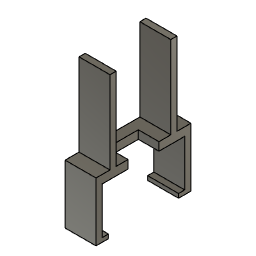
assembly v45 (Autodesk Fusion 360 archive; units mm, degrees)
design "bottom clip"
Autodesk Fusion 360 part; units mm, degrees
sketch "Sketch1" plane through (0, 0, 0) normal (1, 0, 0) x (0, 1, 0)
  line L0 (0, 0) -> (8, 0)
  line L1 (8, 0) -> (8, -9)
  line L2 (8, -9) -> (6.8, -9)
  line L3 (6.8, -9) -> (6.8, -9.8)
  line L4 (6.8, -9.8) -> (9.2, -9.8)
  line L5 (9.2, -9.8) -> (9.2, 1.6)
  line L6 (9.2, 1.6) -> (6.5, 1.6)
  line L7 (6.5, 1.6) -> (6.5, 17.6)
  line L8 (6.5, 17.6) -> (5.3, 17.6)
  line L9 (5.3, 17.6) -> (5.3, 1.6)
  line L10 (5.3, 1.6) -> (0, 1.6)
  line L11 (0, 1.6) -> (0, 0)
  dimension "d1" = 1.2
  dimension "d2" = 1.2
  dimension "d3" = 1.6
  dimension "d4" = 8
  dimension "d6" = 0.8
  dimension "d7" = 1.2
  dimension "d8" = 16
  dimension "d9" = 5.3
  dimension "d17" = 9
  constraint coincident L0.start L11.end
  constraint horizontal L0
  constraint perpendicular L0 L1
  constraint perpendicular L1 L2
  constraint perpendicular L2 L3
  constraint perpendicular L1 L4
  constraint perpendicular L4 L5
  constraint perpendicular L5 L6
  constraint perpendicular L6 L7
  constraint perpendicular L7 L8
  constraint perpendicular L6 L9
  constraint perpendicular L9 L10
  constraint perpendicular L0 L11
  constraint collinear L6 L10
  measures "d1" distance of L1 L5
  measures "d2" distance of L7 L9
  measures "d3" distance of L0 L10
  measures "d4" distance of L0.start L0.end
  measures "d6" distance of L2.end L3.end
  measures "d7" distance of L1.end L2.end
  measures "d8" distance of L6.end L7.end
  measures "d9" distance of L9.end L10.end
  measures "d17" distance of L0.end L1.end
extrude "Extrude1" add sketch "Sketch1" along normal blind 6
sketch "Sketch2" plane through (0, 0, 1.6) normal (0, 0, 1) x (-1, 0, 0)
  line L0 (0, -5.3) -> (0, 0)
  line L1 (0, 0) -> (-6, 0)
  line L2 (-6, 0) -> (-6, -5.3)
  line L3 (-6, -5.3) -> (0, -5.3)
  line L4 (-6, 0) -> (-2, 0)
  line L5 (-2, 0) -> (-2, -3)
  line L6 (-2, -3) -> (-6, -3)
  line L7 (-6, -3) -> (-6, 0)
  dimension "d12" = 4
  dimension "d13" = 3
  constraint horizontal L4
  constraint vertical L5
  constraint horizontal L6
  constraint vertical L7
  constraint coincident L1.end L2.start
  measures "d12" distance of L5.end L6.end
  measures "d13" distance of L1.end L6.end
extrude "Extrude2" cut sketch "Sketch2" against normal through all contours L1 L2 L4 L5 L6 L7
mirror "Mirror1" about plane through (0, 0, 0) normal (0, 1, 0) of bodies 1 merged

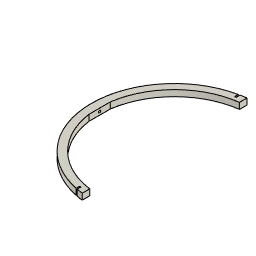
design "midRing"
Autodesk Fusion 360 part; units mm, degrees
sketch "Sketch1" plane through (0, 0, 0) normal (0, 0, 1) x (1, 0, 0)
  circle A0 centre (0, 0) radius 100
  circle A1 centre (0, 0) radius 105
  circle A2 centre (0, 0) radius 109.9
  line L0 (0, 0) -> (0, -109.9) construction
  line L1 (0, 0) -> (109.9, 0) construction
  line L2 (13, -99.1514) -> (13, -109.1284)
  line L3 (-13, -99.1514) -> (-13, -109.1284)
  circle A3 centre (-18, -103.4456) radius 1.5
  circle A4 centre (-28, -101.1978) radius 1.5
  line L4 (-13, 99.1514) -> (-13, 109.1284)
  line L5 (13, 99.1514) -> (13, 109.1284)
  circle A5 centre (-18, 103.4456) radius 1.5
  circle A6 centre (-28, 101.1978) radius 1.5
  line L6 (-22.7, -107.5301) -> (-22.7, -102.875)
  line L7 (-22.7, -102.875) -> (-21, -102.875)
  line L8 (-21, -102.875) -> (-21, -107.875)
  line L9 (-22.7, 107.5301) -> (-22.7, 102.875)
  line L10 (-21, 102.875) -> (-21, 107.875)
  line L11 (-22.7, 102.875) -> (-21, 102.875)
  line L12 (-99, 14.1067) -> (-99, -14.1067)
  line L13 (-100, 0) -> (0, 0) construction
  dimension "d1" = 200
  dimension "d2" = 5
  dimension "d3" = 9.9
  dimension "d4" = 26
  dimension "d5" = 5
  dimension "d7" = 3
  dimension "d8" = 3
  dimension "d9" = 10
  dimension "d21" = 8
  dimension "d22" = 1.7
  dimension "d23" = 5
  dimension "d24" = 1
  constraint coincident A0.centre A1.centre
  constraint concentric A0 A1
  constraint coincident A2 L0.end
  constraint vertical L0
  constraint coincident A2 L1.end
  constraint perpendicular L0 L1
  constraint coincident A0 L2.start
  constraint coincident A2 L2.end
  constraint perpendicular L1 L2
  constraint coincident A0 L3.start
  constraint coincident A2 L3.end
  constraint parallel L2 L3
  constraint equal L2 L3
  constraint coincident A1 A3.centre
  constraint coincident A1 A4.centre
  constraint symmetric L1 L2.start L5.start
  constraint symmetric L1 L2.end L5.end
  constraint symmetric L1 L3.start L4.start
  constraint symmetric L1 L3.end L4.end
  constraint symmetric L1 A3 A5
  constraint symmetric L1 A4 A6
  constraint coincident A2 L6.start
  constraint vertical L6
  constraint perpendicular L6 L7
  constraint coincident A2 L8.end
  constraint perpendicular L7 L8
  constraint symmetric L1 L6.start L9.start
  constraint symmetric L1 L6.end L9.end
  constraint symmetric L1 L7.end L10.start
  constraint symmetric L1 L8.end L10.end
  constraint coincident A0 L12.start
  constraint coincident A0 L12.end
  constraint vertical L12
  constraint coincident A0 L13.start
  constraint perpendicular L0 L13
  measures "d1" diameter of A0
  measures "d2" distance of A0 A1
  measures "d3" distance of A0 A2
  measures "d4" distance of L2 L3
  measures "d5" distance of L3 A3.centre
  measures "d7" diameter of A4
  measures "d8" diameter of A3
  measures "d9" horizontal distance of A3.centre A4.centre
  measures "d21" distance of L3 L8
  measures "d22" distance of L6.end L7.end
  measures "d23" distance of L7.end L8.end
  measures "d24" distance of L12 L13.start
extrude "Extrude1" add sketch "Sketch1" along normal mid plane 8.1 contours A0 A1 L3 A3 A4 L4 A5 A6 L7 L8 L10 L11 | A0 L12 | A1 A2 L4 A5 L10 | A1 A2 L3 A3 L8 | A1 A5 | A1 A5 | A1 A3 | A1 A3 | A1 A2 A4 A6 L6 L7 L9 L11 | A1 A6 | A1 A6 | A1 A4 | A1 A4 picked at (-99.2962, 1.5721)
ref_plane "WorkPlane1" through (-110, 0, 0) normal (1, 0, 0) x (0, 1, 0)
sketch "Sketch3" plane through (-110, 0, 0) normal (1, 0, 0) x (0, 1, 0)
  circle A0 centre (0, 0) radius 1.55
  dimension "d16" = 3.1
  constraint coincident A0.centre origin
  measures "d16" diameter of A0
extrude "Extrude4" cut sketch "Sketch3" along normal through all

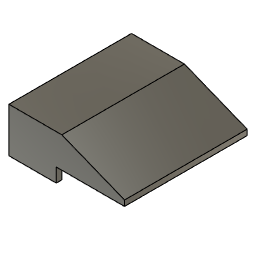
design "top clip"
Autodesk Fusion 360 part; units mm, degrees
sketch "Sketch1" plane through (0, 0, 0) normal (0, 0, 1) x (1, 0, 0)
  line L0 (3, 8) -> (-3, 8)
  line L1 (-3, 8) -> (-3, -8)
  line L2 (-3, -8) -> (3, -8)
  line L3 (3, -8) -> (3, 8)
  line L4 (3, 8) -> (-3, -8) construction
  line L5 (-3, 8) -> (3, -8) construction
  line L6 (3.8, 8.8) -> (-3.8, 8.8)
  line L7 (-3.8, 8.8) -> (-3.8, -8.8)
  line L8 (-3.8, -8.8) -> (3.8, -8.8)
  line L9 (3.8, -8.8) -> (3.8, 8.8)
  line L10 (3.8, 8.8) -> (-3.8, -8.8) construction
  line L11 (-3.8, 8.8) -> (3.8, -8.8) construction
  dimension "d1" = 6
  dimension "d2" = 16
  dimension "d3" = 0.8
  dimension "d4" = 0.8
  constraint horizontal L0
  constraint perpendicular L0 L1
  constraint parallel L0 L2
  constraint parallel L1 L3
  constraint coincident L4 origin
  constraint coincident L5 origin
  constraint horizontal L6
  constraint perpendicular L6 L7
  constraint parallel L6 L8
  constraint parallel L7 L9
  constraint coincident L10 origin
  constraint coincident L11 origin
  measures "d1" distance of L0.start L0.end
  measures "d2" distance of L0.start L2.end
  measures "d3" distance of L0 L6
  measures "d4" distance of L3 L9
extrude "Extrude1" add sketch "Sketch1" along normal blind 0.4 contours L0 L1 L2 L3 | L6 L7 L8 L9
extrude "Extrude2" add sketch "Sketch1" against normal blind 6
sketch "Sketch2" plane through (0, 0, 0) normal (0, 1, 0) x (1, 0, 0)
  line L0 (-3.8, 6) -> (3.8, 6)
  line L1 (3.8, 4) -> (12.8, 4)
  line L2 (12.8, 4) -> (12.8, 3.2)
  line L3 (3.8, 0) -> (-3.8, 0)
  line L4 (12.8, 3.2) -> (3.8, -0.4)
  line L5 (3.8, -0.4) -> (3.8, 4)
  line L6 (3.8, -0.4) -> (3.8, 6)
  point P0 (3, 0)
  point P1 (3.8, -0.4)
  dimension "d9" = 0.8
  dimension "d10" = 4
  dimension "d15" = 9
  constraint perpendicular L1 L2
  constraint coincident P1 L4.end
  constraint coincident L1.start L5.end
  constraint coincident L1.start L6
  measures "d9" distance of L1.end L2.end
  measures "d10" distance of L1 L3
  measures "d15" distance of L1.start L1.end
extrude "Extrude3" add sketch "Sketch2" along normal mid plane 17.6
sketch "Sketch3" plane through (0, 0, -6) normal (0, 0, -1) x (1, 0, 0)
  line L0 (3, 8) -> (3, -8)
  line L1 (3, -8) -> (-3, -8)
  line L2 (-3, -8) -> (-3, 8)
  line L3 (-3, 8) -> (3, 8)
  line L4 (3.8, -8.8) -> (3.8, 8.8)
  line L5 (3.8, 8.8) -> (-3.8, 8.8)
  line L6 (-3.8, 8.8) -> (-3.8, -8.8)
  line L7 (-3.8, -8.8) -> (3.8, -8.8)
  line L8 (3.8, 8.8) -> (3, 8.8)
  line L9 (3, 8.8) -> (3, -8.8)
  line L10 (3, -8.8) -> (3.8, -8.8)
  line L11 (3.8, -8.8) -> (3.8, 8.8)
  line L12 (3, 8) -> (3, -8)
  constraint horizontal L8
  constraint vertical L9
  constraint horizontal L10
  constraint vertical L11
  constraint coincident L7 L9.end
  constraint coincident L4.end L5.start
  constraint coincident L9 L0.end
extrude "Extrude4" cut sketch "Sketch3" against normal blind 2 contours L0 L4 L5 L7 L8 L9 L10 L11 L12

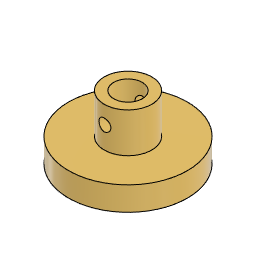
design "tripod attachement thin"
Autodesk Fusion 360 part; units mm, degrees
sketch "Sketch1" plane through (0, 0, 0) normal (0, 0, 1) x (1, 0, 0)
  circle A0 centre (0, 0) radius 6
  circle A1 centre (0, 0) radius 11
  line L0 (-9.7723, 5.05) -> (-3.24, 5.05)
  line L1 (-9.7723, -5.05) -> (-3.24, -5.05)
  line L2 (3.24, 5.05) -> (9.7723, 5.05)
  line L3 (3.24, -5.05) -> (9.7723, -5.05)
  line L4 (0, 0) -> (-6, 0) construction
  circle A2 centre (0, 0) radius 15
  dimension "d1" = 12
  dimension "d2" = 22
  dimension "d3" = 10.1
  dimension "d4" = 10.1
  dimension "d17" = 4
  constraint coincident A0.centre A1.centre
  constraint coincident A1 L0.start
  constraint coincident A0 L0.end
  constraint horizontal L0
  constraint coincident A1 L1.start
  constraint coincident A0 L1.end
  constraint parallel L0 L1
  constraint coincident A0 L2.start
  constraint parallel L0 L2
  constraint coincident A0 L3.start
  constraint parallel L1 L3
  constraint coincident A1 L2.end
  constraint coincident A1 L3.end
  constraint coincident A0 L4.end
  constraint horizontal L4
  constraint symmetric L0 L1 L4
  constraint symmetric L2 L3 L4
  measures "d1" diameter of A0
  measures "d2" diameter of A1
  measures "d3" distance of L0 L1
  measures "d4" distance of L2 L3
  measures "d17" distance of A1 A2
extrude "Extrude1" add sketch "Sketch1" along normal blind 16 contours A0
extrude "Extrude2" add sketch "Sketch1" along normal blind 6 contours A0 A1 L2 L3 | A0 A1 L0 L2 | A0 A1 L1 L3 | A0 A1 L0 L1 | A2
hole "Hole1" at (0, 0, 0) direction (0, 0, 1) diameter 5.118 depth 9 tip angle 180
thread "Thread1" "ANSI Unified Screw Threads 0.25 1/4-20 UNC 1B" major diameter 6.35 minor diameter 5.1181 pitch 1.27 angle 60 modelled right hand crest width 0.3461 on face at (0.1276, 2.5558, 3) crest through (-2.5591, 0, 0.3175)
sketch "Sketch2" plane through (0, 0, 16) normal (0, 0, 1) x (-1, 0, 0)
  circle A0 centre (0, 0) radius 6
  circle A1 centre (0, 0) radius 3.6
  dimension "d18" = 2.4
  constraint concentric A0 A1
  measures "d18" distance of A0 A1
extrude "Extrude3" cut sketch "Sketch2" against normal blind 7 contours A1
sketch "Sketch3" plane through (0, 0, 0) normal (0, 1, 0) x (1, 0, 0)
  line L0 (-6, -6) -> (6, -6)
  line L1 (-6, -16) -> (6, -16)
  circle A0 centre (0, -11.5) radius 1.5
  line L2 (0, -11.5) -> (0, -10) construction
  line L3 (0, -10) -> (0, -6) construction
  dimension "d19" = 4
  dimension "d20" = 3
  constraint coincident A0.centre L2.start
  constraint coincident A0 L2.end
  constraint vertical L2
  constraint midpoint L0 L3.end
  constraint perpendicular L0 L3
  measures "d19" distance of L2.end L3.end
  measures "d20" diameter of A0
extrude "Extrude4" cut sketch "Sketch3" along normal through all and the other way through all

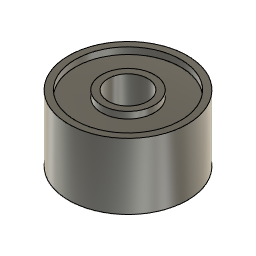
design "3/9 mm bearing"
Autodesk Fusion 360 part; units mm, degrees
sketch "Sketch1" plane through (0, 0, 0) normal (0, 0, 1) x (1, 0, 0)
  circle A0 centre (0, 0) radius 4.5
  circle A1 centre (0, 0) radius 2
  circle A2 centre (0, 0) radius 1.5
  circle A3 centre (0, 0) radius 4
  dimension "d1" = 3
  dimension "d2" = 0.5
  dimension "d3" = 0.5
  dimension "d4" = 9
  constraint coincident A0.centre A1.centre
  constraint concentric A0 A1
  measures "d1" diameter of A2
  measures "d2" distance of A1 A2
  measures "d3" distance of A0 A3
  measures "d4" diameter of A0
extrude "Extrude1" add sketch "Sketch1" against normal blind 5 contours A0 | A1 | A2 | A3
extrude "Extrude2" cut sketch "Sketch1" against normal blind 0.5 contours A3
extrude "Extrude3" cut sketch "Sketch1" against normal through all contours A2

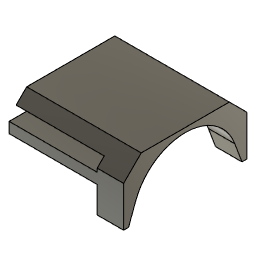
design "plate clip"
Autodesk Fusion 360 part; units mm, degrees
sketch "Sketch1" plane through (0, 0, 0) normal (1, 0, 0) x (0, 1, 0)
  line L0 (0, 0) -> (0, 10) construction
  circle A0 centre (0, 10) radius 6
  line L1 (0, 10) -> (0, 15.3) construction
  line L2 (9, 0) -> (-9, 0) construction
  line L3 (-9, 0) -> (-9, 3) construction
  line L4 (-9, 3) -> (9, 3) construction
  line L5 (9, 3) -> (9, 0) construction
  line L6 (9, 0) -> (-9, 3) construction
  line L7 (-9, 0) -> (9, 3) construction
  line L8 (9, 3) -> (5.6247, 12.0888)
  line L9 (-9, 3) -> (-5.6247, 12.0888) construction
  line L10 (0, 10) -> (0, 14) construction
  line L11 (0, 16.5) -> (7, 16.5)
  line L12 (7, 16.5) -> (7, 12.9)
  line L13 (7, 12.9) -> (5.2526, 12.9)
  line L14 (7, 14.1) -> (4.3806, 14.1)
  line L15 (7, 15.3) -> (2.8125, 15.3)
  line L16 (7, 12.9) -> (7, 9.9)
  line L17 (7, 9.9) -> (6.4375, 9.9)
  line L18 (0, 16) -> (0, 16.5)
  point P0 (0, 1.5)
  dimension "d2" = 12
  dimension "d3" = 5.3
  dimension "d4" = 3
  dimension "d5" = 18
  dimension "d6" = 7
  dimension "d7" = 1.2
  dimension "d8" = 1.2
  dimension "d9" = 1.2
  dimension "d10" = 7
  dimension "d11" = 3
  constraint coincident L0.start origin
  constraint vertical L0
  constraint coincident L0.end A0.centre
  constraint parallel L0 L1
  constraint horizontal L2
  constraint perpendicular L2 L3
  constraint parallel L2 L4
  constraint parallel L3 L5
  constraint coincident L6 P0
  constraint coincident L7 P0
  constraint coincident L0 P0
  constraint coincident A0 L8.end
  constraint tangent A0 L8
  constraint coincident A0 L9.end
  constraint tangent A0 L9
  constraint coincident L0.start L2
  constraint coincident L1 L10.end
  constraint parallel L1 L10
  constraint perpendicular L1 L11
  constraint perpendicular L11 L12
  constraint perpendicular L12 L13
  constraint coincident L12 L14.start
  constraint perpendicular L12 L14
  constraint coincident L12 L15.start
  constraint coincident A0 L15.end
  constraint perpendicular L12 L15
  constraint coincident L1.end L15
  constraint coincident A0 L14.end
  constraint coincident A0 L13.end
  constraint perpendicular L13 L16
  constraint coincident L8 L17.end
  constraint perpendicular L16 L17
  constraint parallel L1 L18
  constraint coincident L11.start L18.end
  constraint coincident A0 L18.start
  constraint collinear L1 L18
  measures "d2" diameter of A0
  measures "d3" distance of L0.end L1.end
  measures "d4" distance of L2.start L4.end
  measures "d5" distance of L2.start L2.end
  measures "d6" distance of L0.end L4
  measures "d7" distance of L14 L15
  measures "d8" distance of L11 L15
  measures "d9" distance of L13 L14
  measures "d10" distance of L1 L12
  measures "d11" distance of L12.end L16.end
extrude "Extrude1" add sketch "Sketch1" along normal blind 3 contours A0 L8 L13 L16 L17 | A0 L11 L12 L15 L18 | A0 L12 L13 L14 | A0 L12 L14 L15
extrude "Extrude2" add sketch "Sketch1" against normal blind 10 contours A0 L11 L12 L15 L18 | A0 L12 L13 L14
mirror "Mirror1" about plane through (0, 0, 0) normal (0, 1, 0) of bodies 1 merged
chamfer "Chamfer1" distance 2 angle 45 2 edges at (-3.5, -7, 16.5) (-3.5, 7, 16.5)

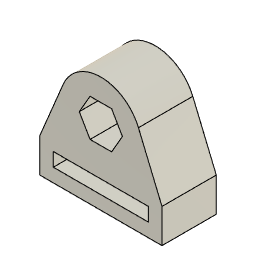
design "inner connector V2 7mm base drone"
Autodesk Fusion 360 part; units mm, degrees
sketch "Sketch1" plane through (0, 0, 0) normal (0, 1, 0) x (1, 0, 0)
  line L0 (-9, 0) -> (9, 0)
  line L1 (9, 0) -> (9, -3)
  line L2 (-9, -3) -> (-9, 0)
  line L3 (0, 0) -> (0, -9) construction
  circle A0 centre (0, -9) radius 6
  line L4 (-5.5385, -11.3077) -> (-9, -3)
  line L5 (5.5385, -11.3077) -> (9, -3)
  line L6 (1.5877, -11.75) -> (3.1754, -9)
  line L7 (3.1754, -9) -> (1.5877, -6.25)
  line L8 (1.5877, -6.25) -> (-1.5877, -6.25)
  line L9 (-1.5877, -6.25) -> (-3.1754, -9)
  line L10 (-3.1754, -9) -> (-1.5877, -11.75)
  line L11 (-1.5877, -11.75) -> (1.5877, -11.75)
  line L12 (-7, 0) -> (-7, -2)
  line L13 (-7, -2) -> (7, -2)
  line L14 (7, -2) -> (7, 0)
  line L15 (9, 0) -> (9, 2)
  line L16 (9, 2) -> (-9, 2)
  line L17 (-9, 2) -> (-9, 0)
  circle A1 centre (-5, -9.4) radius 0.5
  line L18 (-5.9867, -9.4) -> (5.9867, -9.4) construction
  circle A2 centre (5, -9.4) radius 0.5
  point P0 (0, -9)
  dimension "d3" = 3
  dimension "d4" = 12
  dimension "d6" = 5.5
  dimension "d10" = 2
  dimension "d11" = 14
  dimension "d12" = 2
  dimension "d24" = 2
  dimension "d25" = 7
  dimension "d26" = 10
  dimension "d27" = 1
  dimension "d28" = 0.4
  constraint horizontal L0
  constraint perpendicular L0 L1
  constraint coincident L3.start origin
  constraint perpendicular L0 L3
  constraint coincident L3.start L0
  constraint vertical L2
  constraint coincident A0 L4.start
  constraint coincident A0 L5.start
  constraint tangent A0 L4
  constraint tangent A0 L5
  constraint equal L1 L2
  constraint coincident P0 L3.end
  constraint parallel L3 L12
  constraint perpendicular L12 L13
  constraint coincident L0 L14.end
  constraint perpendicular L0 L14
  constraint coincident L0 L12.start
  constraint symmetric L3 L12 L14
  constraint perpendicular L0 L15
  constraint perpendicular L15 L16
  constraint vertical L17
  constraint horizontal L11
  constraint coincident A0 L18.start
  constraint coincident A0 L18.end
  constraint horizontal L18
  constraint coincident A1.centre L18
  constraint coincident L18 A2.centre
  constraint symmetric L3 A1 A2
  measures "d3" distance of L0.end L1.end
  measures "d4" diameter of A0
  measures "d6" distance of L6 L9
  measures "d10" distance of L12.start L12.end
  measures "d11" distance of L12 L14
  measures "d12" distance of L2 L12
  measures "d24" distance of L0.start L16.end
  measures "d25" distance of P0 L13
  measures "d26" distance of A1.centre A2.centre
  measures "d27" diameter of A1
  measures "d28" distance of P0 L18
extrude "Extrude1" add sketch "Sketch1" along normal mid plane 8 contours L0 L15 L16 L17 | L0 L1 L2 A0 L4 L5 L12 L13 L14 | A0 | A1 | A2

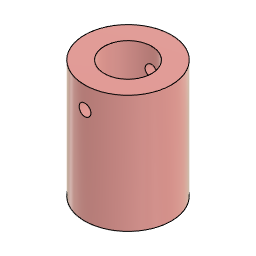
design "Base core V2 thin"
Autodesk Fusion 360 part; units mm, degrees
sketch "Sketch1" plane through (0, 0, 0) normal (0, 1, 0) x (1, 0, 0)
  line L0 (0, -30) -> (6.025, -30) construction
  line L1 (0, 0) -> (0, -30) construction
  line L2 (6.025, -30) -> (11.025, -30)
  line L3 (11.025, -30) -> (11.025, 0)
  line L4 (6.025, -30) -> (6.025, -8)
  line L5 (6.025, -8) -> (4.025, -8)
  line L6 (4.025, -4) -> (6.025, -4)
  line L7 (4.025, -8) -> (4.025, -4)
  line L8 (0, 0) -> (6.025, 0) construction
  line L9 (6.025, -4) -> (6.025, 0)
  line L10 (6.025, 0) -> (11.025, 0)
  line L11 (6.025, -12) -> (11.025, -12) construction
  line L12 (11.025, -18) -> (6.025, -18) construction
  dimension "d2" = 6.025
  dimension "d3" = 22
  dimension "d4" = 2
  dimension "d5" = 4
  dimension "d6" = 5
  dimension "d8" = 4
  dimension "d15" = 4
  dimension "d16" = 6
  constraint horizontal L0
  constraint coincident L1.start L8.start
  constraint perpendicular L0 L1
  constraint parallel L0 L2
  constraint perpendicular L0 L3
  constraint perpendicular L0 L4
  constraint perpendicular L4 L5
  constraint perpendicular L6 L7
  constraint vertical L7
  constraint equal L5 L6
  constraint perpendicular L8 L9
  constraint horizontal L8
  constraint coincident L8.end L9.end
  constraint perpendicular L3 L10
  constraint coincident L4 L11.start
  constraint coincident L3 L11.end
  constraint perpendicular L3 L11
  constraint coincident L3 L12.start
  constraint coincident L4 L12.end
  constraint perpendicular L4 L12
  measures "d2" distance of L0.start L0.end
  measures "d3" distance of L0.end L4.end
  measures "d4" distance of L4.end L5.end
  measures "d5" distance of L5.end L6.start
  measures "d6" distance of L0.end L2.end
  measures "d8" distance of L6.end L8.end
  measures "d15" distance of L5 L11
  measures "d16" distance of L11 L12
revolve "Revolve1" add sketch "Sketch1" angle 360 about axis through (0, 0, 0) along (0, 0, 1)
sketch "Sketch3" plane through (0, 0, 0) normal (0, 1, 0) x (1, 0, 0)
  line L0 (-11.025, -30) -> (11.025, -30)
  circle A0 centre (0, -24.5) radius 1.5
  line L1 (0, -24.5) -> (0, -26) construction
  line L2 (0, -26) -> (0, -30) construction
  dimension "d17" = 4
  dimension "d18" = 3
  constraint coincident A0.centre L1.start
  constraint coincident A0 L1.end
  constraint perpendicular L0 L1
  constraint midpoint L0 L2.end
  constraint perpendicular L0 L2
  measures "d17" distance of L1.end L2.end
  measures "d18" diameter of A0
extrude "Extrude2" cut sketch "Sketch3" along normal through all and the other way through all

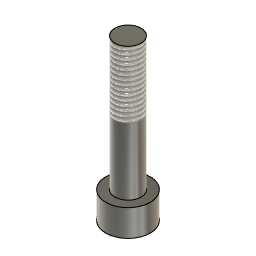
design "din 912 m6"
Autodesk Fusion 360 part; units mm, degrees
sketch "Sketch1" plane through (0, 0, 0) normal (0, 1, 0) x (1, 0, 0)
  line L0 (0, 0) -> (5, 0)
  line L1 (5, 0) -> (5, -6)
  line L2 (5, -6) -> (3, -6)
  line L3 (3, -6) -> (3, -36)
  line L4 (3, -36) -> (0, -36)
  line L5 (0, -36) -> (0, 0)
  dimension "d1" = 3
  dimension "d2" = 5
  dimension "d3" = 6
  dimension "d5" = 30
  constraint coincident L0.start L5.end
  constraint horizontal L0
  constraint perpendicular L0 L1
  constraint perpendicular L1 L2
  constraint perpendicular L0 L3
  constraint perpendicular L3 L4
  constraint perpendicular L4 L5
  measures "d1" distance of L3.end L4.end
  measures "d2" distance of L0.start L0.end
  measures "d3" distance of L0.end L1.end
  measures "d5" distance of L2 L4
revolve "Revolve1" add sketch "Sketch1" angle 360 about axis through (0, 0, 36) along (0, 0, -1)
thread "Thread1" "ISO Metric profile 6.0 M6x1 6g" major diameter 5.884 minor diameter 4.7435 pitch 1 angle 60 resizes the face on face at (2.9851, 0.2987, 26) from (0, 0, 21) to (0, 0, 36)

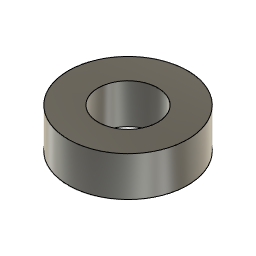
design "6 12 bearing"
Autodesk Fusion 360 part; units mm, degrees
sketch "Sketch1" plane through (0, 0, 0) normal (0, 0, 1) x (1, 0, 0)
  circle A0 centre (0, 0) radius 3
  circle A1 centre (0, 0) radius 6
  dimension "d1" = 12
  dimension "d2" = 6
  constraint coincident A0.centre A1.centre
  constraint concentric A0 A1
  measures "d1" diameter of A1
  measures "d2" diameter of A0
extrude "Extrude1" add sketch "Sketch1" along normal blind 4

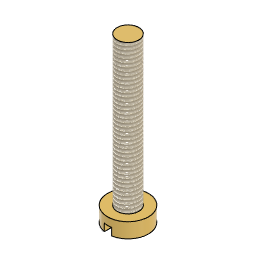
design "20mm M3 slotted screw"
Autodesk Fusion 360 part; units mm, degrees
sketch "Sketch2" plane through (0, 0, 0) normal (0, 1, 0) x (1, 0, 0)
  line L0 (0, 0) -> (2.75, 0)
  line L1 (2.75, 0) -> (2.75, -2)
  line L2 (2.75, -2) -> (1.5, -2)
  line L3 (1.5, -2) -> (1.5, -22)
  line L4 (1.5, -22) -> (0, -22)
  line L5 (0, -22) -> (0, 0)
  dimension "d1" = 2
  dimension "d2" = 20
  dimension "d3" = 1.5
  dimension "d4" = 2.75
  constraint coincident L0.start L5.end
  constraint horizontal L0
  constraint perpendicular L0 L1
  constraint perpendicular L1 L2
  constraint perpendicular L2 L3
  constraint perpendicular L3 L4
  constraint perpendicular L0 L5
  measures "d1" distance of L0.end L1.end
  measures "d2" distance of L2.end L3.end
  measures "d3" distance of L3.end L4.end
  measures "d4" distance of L0.start L0.end
revolve "Revolve1" add sketch "Sketch2" angle 360 about axis through (0, 0, 22) along (0, 0, -1)
thread "Thread1" "ISO Metric profile 3.0 M3x0.5 6g" major diameter 2.927 minor diameter 2.3555 pitch 0.5 angle 60 resizes the face on face at (1.4925, 0.1494, 15.3333)
sketch "Sketch3" plane through (0, 0, 0) normal (0, 0, -1) x (1, 0, 0)
  circle A0 centre (0, 0) radius 2.75
  line L0 (-0.5, -2.7042) -> (-0.5, 2.7042)
  line L1 (0.5, -2.7042) -> (0.5, 2.7042)
  dimension "d6" = 1
  constraint coincident A0 L0.start
  constraint coincident A0 L0.end
  constraint vertical L0
  constraint coincident A0 L1.start
  constraint coincident A0 L1.end
  constraint parallel L0 L1
  constraint equal L0 L1
  measures "d6" distance of L0 L1
extrude "Extrude1" cut sketch "Sketch3" against normal blind 1 contours A0 L0 L1
equation "d4 = ( 5.5 / 2 ) * 1 mm"

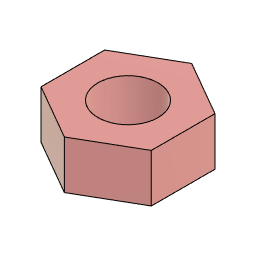
design "M3 DIN934"
Autodesk Fusion 360 part; units mm, degrees
sketch "Sketch1" plane through (0, 0, 0) normal (0, 0, 1) x (1, 0, 0)
  line L0 (2.75, 1.5877) -> (0, 3.1754)
  line L1 (0, 3.1754) -> (-2.75, 1.5877)
  line L2 (-2.75, 1.5877) -> (-2.75, -1.5877)
  line L3 (-2.75, -1.5877) -> (0, -3.1754)
  line L4 (0, -3.1754) -> (2.75, -1.5877)
  line L5 (2.75, -1.5877) -> (2.75, 1.5877)
  circle A0 centre (0, 0) radius 1.5
  dimension "d2" = 3
  dimension "d3" = 5.5
  constraint coincident A0.centre origin
  constraint vertical L5
  measures "d2" diameter of A0
  measures "d3" distance of L2 L5
extrude "Extrude1" add sketch "Sketch1" along normal mid plane 2.4
